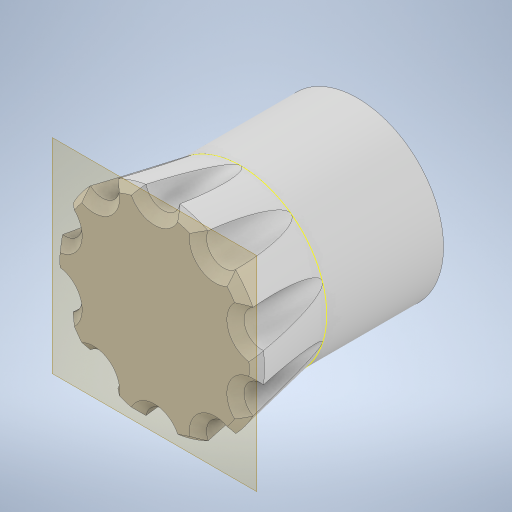
# Autodesk Inventor part: Knob
Saved by Autodesk Inventor 2024.3 (Build 283343000, 343)
## iProperties
Created: 2024-10-19
Part Number: Knob
Material: Generic
Document SubType Name: Modeling
Designer: atrus
Density: 1 g/cm^3
Appearance: Default
Author: atrus
Autodesk Inventor part; units mm, degrees
ref_plane "YZ Plane" through (0, 0, 0) normal (1, 0, 0) x (0, 1, 0)
ref_plane "XZ Plane" through (0, 0, 0) normal (0, 1, 0) x (-1, 0, 0)
ref_plane "XY Plane" through (0, 0, 0) normal (0, 0, 1) x (1, 0, 0)
ref_plane "Work Plane1" through (0, 0, 0.2032) normal (0, 0, 1) x (1, 0, 0)
sketch "Sketch1" plane through (0, 0, 0.2032) normal (0, 0, 1) x (1, 0, 0)
  arc A0 (-2.300112, 1.5) -> (2.300112, 1.5) centre (0, 0) ccw
  line L0 (2.300112, 1.5) -> (-2.300112, 1.5)
  arc A1 (-2.457258, 1.8) -> (2.457258, 1.8) centre (0, 0) ccw
  line L1 (-2.457258, 1.8) -> (2.457258, 1.8)
  circle A2 centre (0, 0) radius 5
  circle A3 centre (0, 0) radius 6
  point P0 (0, 0)
  dimension "d0" = 0.3
  dimension "d1" = 1
  constraints: 2 centre point, 2 end point, 2 point on circle, 1 coincident, 1 other
  measures "d0" distance between parallel lines of L1 L0
  measures "d1" radial gap between concentric circles of A3 A2
ref_plane "Work Plane2" through (-2.746, -2.746, 7) normal (0, 0, 1) x (1, 0, 0)
extrude "Extrusion1" add sketch "Sketch1" along normal up to surface (6.7968 mm away) contours A2
sketch "Sketch2" plane through (0, 0, 7) normal (0, 0, 1) x (1, 0, 0)
  circle A0 centre (0, 0) radius 5 projected
  point P0 (0, 0)
ref_plane "Work Plane3" through (0, 0, 12) normal (0, 0, 1) x (1, 0, 0)
sketch "Sketch3" plane through (0, 0, 12) normal (0, 0, 1) x (1, 0, 0)
  circle A0 centre (0, 0) radius 5 construction
  circle A1 centre (0, 0) radius 6
  point P0 (0, 0)
  dimension "d5" = 1
  constraints: 1 centre point
  measures "d5" radial gap between concentric circles of A1 A0
loft "Loft1" add profiles "Sketch3" section 1 edges at (-5, 0, 7)
sketch "Sketch4" plane through (0, 0, 12) normal (0, 0, 1) x (1, 0, 0)
  circle A0 centre (0, 0) radius 6
  circle A1 centre (0, 6) radius 1
  circle A2 centre (-3.526712, 4.854102) radius 1
  circle A3 centre (-5.706339, 1.854102) radius 1
  circle A4 centre (-5.706339, -1.854102) radius 1
  circle A5 centre (-3.526712, -4.854102) radius 1
  circle A6 centre (0, -6) radius 1
  circle A7 centre (3.526712, -4.854102) radius 1
  circle A8 centre (5.706339, -1.854102) radius 1
  circle A9 centre (5.706339, 1.854102) radius 1
  circle A10 centre (3.526712, 4.854102) radius 1
  point P0 (0, 0)
  dimension "d10" = 2
  dimension "d13" = 360
  constraints: 10 centre point, 1 vertical alignment, 22 other
  measures "d10" diameter of A1
extrude "Extrusion2" cut sketch "Sketch4" against normal through all contours A9 A0 | A0 A9 | A8 A0 | A0 A8 | A10 A0 | A0 A10 | A7 A0 | A0 A7 | A1 A0 | A0 A1 | A6 A0 | A0 A6 | A2 A0 | A0 A2 | A5 A0 | A0 A5 | A3 A0 | A0 A3 | A4 A0 | A0 A4
chamfer "Chamfer1" distance 0.5 angle 45 20 edges at (-4.8541, -3.5267, 12) (-6, 0, 12) (-1.8541, -5.7063, 12) (-2.9389, -4.0451, 12) (0, -5, 12) (1.8541, -5.7063, 12) (2.9389, -4.0451, 12) (4.8541, -3.5267, 12) (4.7553, -1.5451, 12) (6, 0, 12) (4.7553, 1.5451, 12) (4.8541, 3.5267, 12) (2.9389, 4.0451, 12) (1.8541, 5.7063, 12) (0, 5, 12) (-1.8541, 5.7063, 12) (-2.9389, 4.0451, 12) (-4.8541, 3.5267, 12) (-4.7553, 1.5451, 12) (-4.7553, -1.5451, 12)
body "Solid1"
